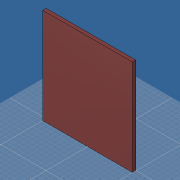
# Autodesk Inventor part: Front_Staubfach
Saved by Autodesk Inventor 2019 (Build 230136000, 136)
## iProperties
Created: 2020-08-04
Part Number: Front_Staubfach
Material: Generisch
Document SubType Name: Modeling
Designer: Stefan
Mass: 3410.85 g
Surface Area: 3721.58 cm^2
Volume: 3410.85 cm^3
Density: 1 g/cm^3
Appearance: Kastanie
Author: Stefan
Autodesk Inventor part; units mm, degrees
ref_plane "YZ Plane" through (0, 0, 0) normal (1, 0, 0) x (0, 1, 0)
ref_plane "XZ Plane" through (0, 0, 0) normal (0, 1, 0) x (-1, 0, 0)
ref_plane "XY Plane" through (0, 0, 0) normal (0, 0, 1) x (1, 0, 0)
sketch "Skizze1" plane through (0, 0, 0) normal (0, 0, 1) x (1, 0, 0)
  line L0 (-199, -212.5) -> (199, -212.5)
  line L1 (199, -212.5) -> (199, 212.5)
  line L2 (199, 212.5) -> (-199, 212.5)
  line L3 (-199, 212.5) -> (-199, -212.5)
  line L4 (-199, -212.5) -> (199, 212.5) construction
  line L5 (199, -212.5) -> (-199, 212.5) construction
  line L6 (182, -195.5) -> (-182, -195.5)
  line L7 (-182, -195.5) -> (-182, 204.5)
  line L8 (-182, 204.5) -> (182, 204.5)
  line L9 (182, 204.5) -> (182, -195.5)
  line L10 (182, -195.5) -> (-182, 204.5) construction
  line L11 (-182, -195.5) -> (182, 204.5) construction
  point P0 (0, 0)
  dimension "d0" = 398
  dimension "d1" = 425
  dimension "d5" = 17
  dimension "d8" = 17
  dimension "d9" = 17
  dimension "d10" = 8
  constraints: 24 end point, 4 parallel, 2 horizontal, 2 midpoint, 2 perpendicular
  measures "d0" distance of L1.end L2.end
  measures "d1" distance of L2.end L0.start
  measures "d5" distance between parallel lines of L1 L9
  measures "d8" distance between parallel lines of L3 L7
  measures "d9" distance between parallel lines of L0 L6
  measures "d10" distance between parallel lines of L2 L8
extrude "Extrusion1" add sketch "Skizze1" along normal blind 15 contours L3 L2 L1 L0 | L6 L7 L8 L9
extrude "Extrusion2" add sketch "Skizze1" against normal blind 6 contours L6 L7 L8 L9
equation "\"d0\" = case_width - 2 * gap_air"
equation "\"d2\" = inner_thickness"
equation "\"d6\" = mdf_thickness"
equation "\"kg_thickness\" = 4.9"
equation "\"ht_thickness\" = 1.9"
equation "\"case_thickness\" = 18"
equation "\"inner_thickness\" = 15"
equation "\"gap_fit\" = 0.1"
equation "\"gap_slide\" = 0.2"
equation "\"gap_air\" = 1"
equation "\"bore_diameter\" = 73"
equation "\"mdf_thickness\" = 6"
equation "\"tape_width\" = 15"
equation "\"tape_thickness\" = 3"
equation "\"inner_depth\" = 255"
equation "\"case_width\" = 400"
